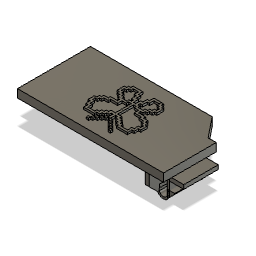
EXL-100-JOYSTICK-BATTERY-COVER (Autodesk Fusion 360 design; units mm, degrees)
Autodesk Fusion 360 part; units mm, degrees
note: some values were not read from the file. Chosen so that the rebuilt part matches the saved one: which face or edge a step refers to.
sketch "Sketch1" plane through (0, 0, 0) normal (0, 1, 0) x (1, 0, 0)
  line L0 (0, -10) -> (-30, -10)
  line L1 (-30, -10) -> (-30, 8)
  line L2 (-30, 8) -> (6, 8)
  line L3 (6, 8) -> (6, -5)
  line L4 (6, -5) -> (4, -5)
  line L5 (4, -5) -> (0, -10)
  dimension "d1" = 30
  dimension "d2" = 18
  dimension "d3" = 36
  dimension "d4" = 13
  dimension "d5" = 2
  constraint horizontal L0
  constraint perpendicular L0 L1
  constraint perpendicular L1 L2
  constraint perpendicular L2 L3
  constraint perpendicular L3 L4
  measures "d1" distance of L0.start L0.end
  measures "d2" distance of L0.end L1.end
  measures "d3" distance of L1.end L2.end
  measures "d4" distance of L2.end L3.end
  measures "d5" distance of L3.end L4.end
extrude "Extrude1" add sketch "Sketch1" along normal blind 1 makes body 1
move_body "Move1" bodies 1 to x (1, 0, 0) y (0, -1, 0) z (0, 0, -1) at (0, 0, -16)
sketch "Sketch2" plane through (0, 0, 0) normal (0, 1, 0) x (1, 0, 0)
  line L0 (105.8333, -439.2083) -> (105.8333, -418.0417)
  line L1 (105.8333, -418.0417) -> (84.6667, -418.0417)
  line L2 (84.6667, -418.0417) -> (84.6667, -460.375)
  line L3 (84.6667, -460.375) -> (107.1563, -460.375)
  line L4 (107.1563, -460.375) -> (107.1563, -481.5417)
  line L5 (107.1563, -481.5417) -> (128.451, -481.5417)
  line L6 (128.451, -481.5417) -> (128.451, -439.2083)
  line L7 (128.451, -439.2083) -> (105.8333, -439.2083)
  line L8 (283.1042, -153.4583) -> (283.1042, -132.2917)
  line L9 (283.1042, -132.2917) -> (330.7292, -132.2917)
  line L10 (330.7292, -132.2917) -> (330.7292, -153.4583)
  line L11 (330.7292, -153.4583) -> (306.9167, -153.4583)
  line L12 (306.9167, -153.4583) -> (306.9167, -174.625)
  line L13 (306.9167, -174.625) -> (264.5833, -174.625)
  line L14 (264.5833, -174.625) -> (264.5833, -153.4583)
  line L15 (264.5833, -153.4583) -> (283.1042, -153.4583)
  line L16 (42.3333, -201.0833) -> (42.3333, -221.787)
  line L17 (42.3333, -221.787) -> (63.5, -221.787)
  line L18 (63.5, -221.787) -> (63.5, -243.4167)
  line L19 (63.5, -243.4167) -> (105.8333, -243.4167)
  line L20 (105.8333, -243.4167) -> (105.8333, -264.5833)
  line L21 (105.8333, -264.5833) -> (174.625, -264.5833)
  line L22 (174.625, -264.5833) -> (174.625, -306.9167)
  line L23 (174.625, -306.9167) -> (216.9583, -306.9167)
  line L24 (216.9583, -306.9167) -> (216.9583, -328.0833)
  line L25 (216.9583, -328.0833) -> (243.4167, -328.0833)
  line L26 (243.4167, -328.0833) -> (243.4167, -174.625)
  line L27 (243.4167, -174.625) -> (201.0833, -174.625)
  line L28 (201.0833, -174.625) -> (201.0833, -153.4583)
  line L29 (201.0833, -153.4583) -> (177.2708, -153.4583)
  line L30 (177.2708, -153.4583) -> (177.2708, -132.2917)
  line L31 (177.2708, -132.2917) -> (224.8958, -132.2917)
  line L32 (224.8958, -132.2917) -> (224.8958, -153.4583)
  line L33 (224.8958, -153.4583) -> (243.4167, -153.4583)
  line L34 (243.4167, -153.4583) -> (243.4167, -105.8333)
  line L35 (243.4167, -105.8333) -> (264.5833, -105.8333)
  line L36 (264.5833, -105.8333) -> (264.5833, -328.0833)
  line L37 (264.5833, -328.0833) -> (291.0417, -328.0833)
  line L38 (291.0417, -328.0833) -> (291.0417, -306.9167)
  line L39 (291.0417, -306.9167) -> (333.375, -306.9167)
  line L40 (333.375, -306.9167) -> (333.375, -264.5833)
  line L41 (333.375, -264.5833) -> (402.1667, -264.5833)
  line L42 (402.1667, -264.5833) -> (402.1667, -243.4167)
  line L43 (402.1667, -243.4167) -> (444.5, -243.4167)
  line L44 (444.5, -243.4167) -> (444.5, -221.787)
  line L45 (444.5, -221.787) -> (465.6667, -221.787)
  line L46 (465.6667, -221.787) -> (465.6667, -201.0833)
  line L47 (465.6667, -201.0833) -> (486.8333, -201.0833)
  line L48 (486.8333, -201.0833) -> (486.8333, -174.625)
  line L49 (486.8333, -174.625) -> (465.6667, -174.625)
  line L50 (465.6667, -174.625) -> (465.6667, -132.2917)
  line L51 (465.6667, -132.2917) -> (444.5, -132.2917)
  line L52 (444.5, -132.2917) -> (444.5, -89.9583)
  line L53 (444.5, -89.9583) -> (465.6667, -89.9583)
  line L54 (465.6667, -89.9583) -> (465.6667, -111.125)
  line L55 (465.6667, -111.125) -> (486.8333, -111.125)
  line L56 (486.8333, -111.125) -> (486.8333, -153.4583)
  line L57 (486.8333, -153.4583) -> (508, -153.4583)
  line L58 (508, -153.4583) -> (508, -216.9583)
  line L59 (508, -216.9583) -> (486.8333, -216.9583)
  line L60 (486.8333, -216.9583) -> (486.8333, -242.4906)
  line L61 (486.8333, -242.4906) -> (465.6667, -242.4906)
  line L62 (465.6667, -242.4906) -> (465.6667, -264.5833)
  line L63 (465.6667, -264.5833) -> (423.3333, -264.5833)
  line L64 (423.3333, -264.5833) -> (423.3333, -285.75)
  line L65 (423.3333, -285.75) -> (354.5417, -285.75)
  line L66 (354.5417, -285.75) -> (354.5417, -306.9167)
  line L67 (354.5417, -306.9167) -> (375.7083, -306.9167)
  line L68 (375.7083, -306.9167) -> (375.7083, -328.0833)
  line L69 (375.7083, -328.0833) -> (396.875, -328.0833)
  line L70 (396.875, -328.0833) -> (396.875, -349.25)
  line L71 (396.875, -349.25) -> (423.3333, -349.25)
  line L72 (423.3333, -349.25) -> (423.3333, -370.4167)
  line L73 (423.3333, -370.4167) -> (444.5, -370.4167)
  line L74 (444.5, -370.4167) -> (444.5, -439.2083)
  line L75 (444.5, -439.2083) -> (423.3333, -439.2083)
  line L76 (423.3333, -439.2083) -> (423.3333, -391.5833)
  line L77 (423.3333, -391.5833) -> (400.8438, -391.5833)
  line L78 (400.8438, -391.5833) -> (400.8438, -370.4167)
  line L79 (400.8438, -370.4167) -> (378.3542, -370.4167)
  line L80 (378.3542, -370.4167) -> (378.3542, -349.25)
  line L81 (378.3542, -349.25) -> (354.5417, -349.25)
  line L82 (354.5417, -349.25) -> (354.5417, -328.0833)
  line L83 (354.5417, -328.0833) -> (306.9167, -328.0833)
  line L84 (306.9167, -328.0833) -> (306.9167, -349.25)
  line L85 (306.9167, -349.25) -> (285.75, -349.25)
  line L86 (285.75, -349.25) -> (285.75, -370.4167)
  line L87 (285.75, -370.4167) -> (306.9167, -370.4167)
  line L88 (306.9167, -370.4167) -> (306.9167, -418.0417)
  line L89 (306.9167, -418.0417) -> (328.0833, -418.0417)
  line L90 (328.0833, -418.0417) -> (328.0833, -460.375)
  line L91 (328.0833, -460.375) -> (379.6771, -460.375)
  line L92 (379.6771, -460.375) -> (379.6771, -439.2083)
  line L93 (379.6771, -439.2083) -> (400.8438, -439.2083)
  line L94 (400.8438, -439.2083) -> (400.8438, -418.0417)
  line L95 (400.8438, -418.0417) -> (423.3333, -418.0417)
  line L96 (423.3333, -418.0417) -> (423.3333, -460.375)
  line L97 (423.3333, -460.375) -> (400.8438, -460.375)
  line L98 (400.8438, -460.375) -> (400.8438, -481.5417)
  line L99 (400.8438, -481.5417) -> (306.9167, -481.5417)
  line L100 (306.9167, -481.5417) -> (306.9167, -439.2083)
  line L101 (306.9167, -439.2083) -> (285.75, -439.2083)
  line L102 (285.75, -439.2083) -> (285.75, -396.875)
  line L103 (285.75, -396.875) -> (264.5833, -396.875)
  line L104 (264.5833, -396.875) -> (264.5833, -349.25)
  line L105 (264.5833, -349.25) -> (243.4167, -349.25)
  line L106 (243.4167, -349.25) -> (243.4167, -396.875)
  line L107 (243.4167, -396.875) -> (222.25, -396.875)
  line L108 (222.25, -396.875) -> (222.25, -439.2083)
  line L109 (222.25, -439.2083) -> (201.0833, -439.2083)
  line L110 (201.0833, -439.2083) -> (201.0833, -481.5417)
  line L111 (201.0833, -481.5417) -> (128.451, -481.5417)
  line L112 (128.451, -481.5417) -> (128.4552, -460.375)
  line L113 (128.4552, -460.375) -> (179.9167, -460.375)
  line L114 (179.9167, -460.375) -> (179.9167, -418.0417)
  line L115 (179.9167, -418.0417) -> (201.0833, -418.0417)
  line L116 (201.0833, -418.0417) -> (201.0833, -370.4167)
  line L117 (201.0833, -370.4167) -> (222.25, -370.4167)
  line L118 (222.25, -370.4167) -> (222.25, -349.25)
  line L119 (222.25, -349.25) -> (201.0833, -349.25)
  line L120 (201.0833, -349.25) -> (201.0833, -328.0833)
  line L121 (201.0833, -328.0833) -> (153.4583, -328.0833)
  line L122 (153.4583, -328.0833) -> (153.4583, -349.25)
  line L123 (153.4583, -349.25) -> (129.6458, -349.25)
  line L124 (129.6458, -349.25) -> (129.6458, -370.4167)
  line L125 (129.6458, -370.4167) -> (107.1562, -370.4167)
  line L126 (107.1563, -370.4167) -> (107.1563, -391.5833)
  line L127 (107.1563, -391.5833) -> (84.6667, -391.5833)
  line L128 (84.6667, -391.5833) -> (84.6667, -439.2083)
  line L129 (84.6667, -439.2083) -> (63.5, -439.2083)
  line L130 (63.5, -439.2083) -> (63.5, -370.4167)
  line L131 (63.5, -370.4167) -> (84.6667, -370.4167)
  line L132 (84.6667, -370.4167) -> (84.6667, -349.25)
  line L133 (84.6667, -349.25) -> (111.125, -349.25)
  line L134 (111.125, -349.25) -> (111.125, -328.0833)
  line L135 (111.125, -328.0833) -> (132.2917, -328.0833)
  line L136 (132.2917, -328.0833) -> (132.2917, -306.9167)
  line L137 (132.2917, -306.9167) -> (153.4583, -306.9167)
  line L138 (153.4583, -306.9167) -> (153.4583, -285.75)
  line L139 (153.4583, -285.75) -> (84.6667, -285.75)
  line L140 (84.6667, -285.75) -> (84.6667, -264.5833)
  line L141 (84.6667, -264.5833) -> (42.3333, -264.5833)
  line L142 (42.3333, -264.5833) -> (42.3333, -242.4906)
  line L143 (42.3333, -242.4906) -> (21.1667, -242.4906)
  line L144 (21.1667, -242.4906) -> (21.1667, -216.9583)
  line L145 (21.1667, -216.9583) -> (0, -216.9583)
  line L146 (0, -216.9583) -> (0, -153.4583)
  line L147 (0, -153.4583) -> (21.1667, -153.4583)
  line L148 (21.1667, -153.4583) -> (21.1667, -111.125)
  line L149 (21.1667, -111.125) -> (42.3333, -111.125)
  line L150 (42.3333, -111.125) -> (42.3333, -89.9583)
  line L151 (42.3333, -89.9583) -> (63.5, -89.9583)
  line L152 (63.5, -89.9583) -> (63.5, -132.2917)
  line L153 (63.5, -132.2917) -> (42.3333, -132.2917)
  line L154 (42.3333, -132.2917) -> (42.3333, -174.625)
  line L155 (42.3333, -174.625) -> (21.1667, -174.625)
  line L156 (21.1667, -174.625) -> (21.1667, -201.0833)
  line L157 (21.1667, -201.0833) -> (42.3333, -201.0833)
  line L158 (359.8333, -89.9583) -> (359.8333, -68.7917)
  line L159 (359.8333, -68.7917) -> (465.6667, -68.7917)
  line L160 (465.6667, -68.7917) -> (465.6667, -89.9583)
  line L161 (465.6667, -89.9583) -> (378.3542, -89.9583)
  line L162 (378.3542, -89.9583) -> (378.3542, -111.125)
  line L163 (378.3542, -111.125) -> (354.5417, -111.125)
  line L164 (354.5417, -111.125) -> (354.5417, -132.2917)
  line L165 (354.5417, -132.2917) -> (306.9167, -132.2917)
  line L166 (306.9167, -132.2917) -> (306.9167, -111.125)
  line L167 (306.9167, -111.125) -> (330.7292, -111.125)
  line L168 (330.7292, -111.125) -> (330.7292, -89.9583)
  line L169 (330.7292, -89.9583) -> (359.8333, -89.9583)
  line L170 (42.3333, -89.9583) -> (129.6458, -89.9583)
  line L171 (129.6458, -89.9583) -> (129.6458, -111.125)
  line L172 (129.6458, -111.125) -> (153.4583, -111.125)
  line L173 (153.4583, -111.125) -> (153.4583, -132.2917)
  line L174 (153.4583, -132.2917) -> (201.0833, -132.2917)
  line L175 (201.0833, -132.2917) -> (201.0833, -111.125)
  line L176 (201.0833, -111.125) -> (177.2708, -111.125)
  line L177 (177.2708, -111.125) -> (177.2708, -89.9583)
  line L178 (177.2708, -89.9583) -> (148.1667, -89.9583)
  line L179 (148.1667, -89.9583) -> (148.1667, -68.7917)
  line L180 (148.1667, -68.7917) -> (42.3333, -68.7917)
  line L181 (42.3333, -68.7917) -> (42.3333, -89.9583)
  line L182 (285.75, -84.6667) -> (264.5833, -84.6667)
  line L183 (264.5833, -84.6667) -> (264.5833, -105.8333)
  line L184 (264.5833, -105.8333) -> (285.75, -105.8333)
  line L185 (285.75, -105.8333) -> (285.75, -84.6667)
  line L186 (243.4167, -84.6667) -> (222.25, -84.6667)
  line L187 (222.25, -84.6667) -> (222.25, -105.8333)
  line L188 (222.25, -105.8333) -> (243.4167, -105.8333)
  line L189 (243.4167, -105.8333) -> (243.4167, -84.6667)
  line L190 (179.9167, -63.5) -> (201.0833, -63.5)
  line L191 (201.0833, -63.5) -> (201.0833, -84.6667)
  line L192 (201.0833, -84.6667) -> (222.25, -84.6667)
  line L193 (222.25, -84.6667) -> (222.25, -63.5)
  line L194 (222.25, -63.5) -> (201.0833, -63.5)
  line L195 (201.0833, -63.5) -> (201.0833, -42.3333)
  line L196 (201.0833, -42.3333) -> (179.9167, -42.3333)
  line L197 (179.9167, -42.3333) -> (179.9167, -63.5)
  line L198 (306.9167, -63.5) -> (285.75, -63.5)
  line L199 (285.75, -63.5) -> (285.75, -84.6667)
  line L200 (285.75, -84.6667) -> (306.9167, -84.6667)
  line L201 (306.9167, -84.6667) -> (306.9167, -63.5)
  line L202 (328.0833, -42.3333) -> (306.9167, -42.3333)
  line L203 (306.9167, -42.3333) -> (306.9167, -63.5)
  line L204 (306.9167, -63.5) -> (328.0833, -63.5)
  line L205 (328.0833, -63.5) -> (328.0833, -42.3333)
  line L206 (179.9167, -21.1667) -> (158.75, -21.1667)
  line L207 (158.75, -21.1667) -> (158.75, -42.3333)
  line L208 (158.75, -42.3333) -> (179.9167, -42.3333)
  line L209 (179.9167, -42.3333) -> (179.9167, -21.1667)
  line L210 (349.25, -21.1667) -> (328.0833, -21.1667)
  line L211 (328.0833, -21.1667) -> (328.0833, -42.3333)
  line L212 (328.0833, -42.3333) -> (349.25, -42.3333)
  line L213 (349.25, -42.3333) -> (349.25, -21.1667)
  line L214 (370.4167, 0) -> (349.25, 0)
  line L215 (349.25, 0) -> (349.25, -21.1667)
  line L216 (349.25, -21.1667) -> (370.4167, -21.1667)
  line L217 (370.4167, -21.1667) -> (370.4167, 0)
  line L218 (158.75, 0) -> (137.5833, 0)
  line L219 (137.5833, 0) -> (137.5833, -21.1667)
  line L220 (137.5833, -21.1667) -> (158.75, -21.1667)
  line L221 (158.75, -21.1667) -> (158.75, 0)
extrude "Extrude2" add sketch "Sketch2" along normal blind 0.5 separate body contours L0 L1 L2 L3 L4 L5 L6 L7 L128 | L2 L14 L16 L17 L18 L19 L20 L21 L22 L23 L24 L25 L26 L27 L28 L29 L30 L31 L32 L33 L34 L35 L36 L37 L38 L39 L40 L41 L42 L43 L44 L45 L46 L47 L48 L49 L50 L51 L52 L53 L54 L55 L56 L57 L58 L59 L60 L61 L62 L63 L64 L65 L66 L67 L68 L69 L70 L71 L72 L73 L74 L75 L96 L97 L98 L99 L100 L101 L102 L103 L104 L105 L106 L107 L108 L109 L110 L111 L112 L113 L114 L115 L116 L117 L118 L119 L120 L121 L122 L123 L124 L125 L126 L127 L128 L129 L130 L131 L132 L133 L134 L135 L136 L137 L138 L139 L140 L141 L142 L143 L144 L145 L146 L147 L148 L149 L150 L151 L152 L153 L154 L155 L156 L157 L161 L170 L174 | L218 L219 L220 L221 | L206 L207 L208 L209 | L190 L195 L196 L197 | L191 L192 L193 L194 | L186 L187 L188 L189 | L214 L215 L216 L217 | L210 L211 L212 L213 | L202 L203 L204 L205 | L198 L199 L200 L201 | L182 L183 L184 L185 | L31 L151 L170 L171 L172 L173 L174 L175 L176 L177 L178 L179 L180 L181 | L8 L9 L10 L11 L12 L13 L14 L15 L36 L165 | L9 L53 L158 L159 L160 L161 L162 L163 L164 L165 L166 L167 L168 L169 makes body 2 at (84.6667, 0.5, 75.8472)
scale "Scale1" factors (0.2, 1, 0.2) about (243.4167, 0, 174.625) bodies 2
move_body "Move2" bodies 2 to x (1, 0, 0) y (0, 1, 0) z (0, 0, 1) at (-239.4762, 0, -125.5632)
scale "Scale2" factors (0.2, 1, 0.2) about (8.1738, 0, 49.0618) bodies 2
move_body "Move3" bodies 2 to x (1, 0, 0) y (0, 1, 0) z (0, 0, 1) at (-21.1687, 0, -68.5097)
scale "Scale3" factors (0.639764, 1, 0.639764) about (-12.995, 0, -19.448) bodies 2
move_body "Move4" bodies 2 to x (1, 0, 0) y (0, 1, 0) z (0, 0, 1) at (0, 0, 23.8705)
move_body "Move5" bodies 2 to x (-1, 0, 0) y (0, 1, 0) z (0, 0, -1) at (-39.5316, 0, 8.7893)
move_body "Align1" bodies 2 to x (1, 0, 0) y (0, 1, 0) z (0, 0, 1) at (14.2658, 0, -18.7938)
box "BoxPrimitive1" add length 5 width 13 height 2 placed x (0, 0, 1) y (1, 0, 0) z (0, 1, 0) at (-45, 0, -5) separate body makes body 3
move_body "Move6" bodies 3 to x (0, 0, 1) y (0, 1, 0) z (-1, 0, 0) at (-50, 0, 40)
move_body "Align2" bodies 3 to x (1, 0, 0) y (0, -1, 0) z (0, 0, -1) at (20, 1, -15.5)
move_body "Move7" bodies 3 to x (1, 0, 0) y (0, 1, 0) z (0, 0, 1) at (0, -2, 0)
move_body "Move8" bodies 3 to x (1, 0, 0) y (0, 1, 0) z (0, 0, 1) at (-2, 0, 0)
chamfer "Chamfer1" distance 2 angle 45 1 edges at (-27, -3, -17) on bodies 3
box "BoxPrimitive2" add length 15 width 1 height 10 placed x (0, 0, 1) y (1, 0, 0) z (0, 1, 0) at (3, 0, -3) separate body makes body 4
move_body "Align3" bodies 4 to x (1, 0, 0) y (0, -1, 0) z (0, 0, -1) at (2, 9, -10)
move_body "Move9" bodies 4 to x (1, 0, 0) y (0, 1, 0) z (0, 0, 1) at (-2, 0, 0)
move_face "MoveFace1" by (0, 0, 1) 1 faces at (3.3333, 5.6667, -22) on bodies 4
move_face "MoveFace2" by (0, 0, -1) 1 faces at (3.3333, 5.6667, -7) on bodies 4
move_body "Move10" bodies 4 to x (1, 0, 0) y (0, 1, 0) z (0, 0, 1) at (0, -10, 0)
box "BoxPrimitive3" add length 2 width 2 height 13 placed x (0, 1, 0) y (-1, 0, 0) z (0, 0, 1) at (6, -11, 0) separate body makes body 5
move_body "Align4" bodies 5 to x (0, 0, 1) y (0, 1, 0) z (-1, 0, 0) at (4, 0, -25)
move_body "Move11" bodies 5 to x (0, 0, -1) y (0, 1, 0) z (1, 0, 0) at (25, 0, -17)
chamfer "Chamfer2" distance 2 angle 45 1 edges at (6, -11, -14.5) on bodies 5
move_body "Move12" bodies 2 to x (1, 0, 0) y (0, 1, 0) z (0, 0, 1) at (0, 1, 0)
move_face "MoveFace3" by (0, 1, 0) 1 faces at (-20, 0, -20) on bodies 1
move_face "MoveFace4" by (0, -2, 0) 1 faces at (3.6667, -1, -12.3333) on bodies 4
move_body "Move13" bodies 4 5 to x (1, 0, 0) y (0, 1, 0) z (0, 0, 1) at (0, 2, 0)
combine "Combine1" operation add target body 1 tool bodies 3 4 5 2 keep tools result as body 6 in component "Component"
move_face "MoveFace5" by (0, -2.5, 0) 1 faces at (3.6667, -1, -12.3333) on bodies 4
move_body "Move14" bodies 4 5 to x (1, 0, 0) y (0, 1, 0) z (0, 0, 1) at (0, 2.5, 0)
sketch "Sketch6" plane through (0, 0, 0) normal (0, 0, 1) x (1, 0, 0)
  line L0 (5.8145, -7.1066) -> (5.8145, -2)
  constraint vertical L0
split "Split1" by curves path "Sketch6" along L0 bodies 5 makes body 7 at (5.9382, -4.5622, -16.6667)
delete_body "RemoveBody1" bodies 7
combine "Combine1'" operation add target body 1 tool bodies 3 4 5 2 keep tools result as body 8 in component "Component'"
copy_body "CopyPasteBodies1" bodies 4 5 makes body 9 makes body 10
move_body "Move15" bodies 9 10 to x (1, 0, 0) y (0, 1, 0) z (0, 0, 1) at (0, 0, 0)
box "BoxPrimitive4" add length 9 width 2 height 2 placed x (0, 0, -1) y (-1, 0, 0) z (0, 1, 0) at (9, 0, -12) separate body makes body 11
move_body "Align5" bodies 11 to x (1, 0, 0) y (0, -1, 0) z (0, 0, -1) at (-1, 3, -31)
move_body "Move16" bodies 11 to x (1, 0, 0) y (0, 1, 0) z (0, 0, 1) at (0, -4, 0)
move_body "Move17" bodies 10 to x (1, 0, 0) y (0, 1, 0) z (0, 0, 1) at (2, 0, 0)
sketch "Sketch8" plane through (0, 0, 0) normal (0, 0, 1) x (1, 0, 0)
cylinder "CylinderPrimitive1" add diameter 3 height 13 placed x (1, 0, 0) y (0, 1, 0) z (0, 0, 1) at (3.5, -7.5, 0) separate body makes body 12
move_body "Move18" bodies 12 to x (1, 0, 0) y (0, 1, 0) z (0, 0, 1) at (0.943, 1.066, 0)
box "BoxPrimitive5" add length 3.884 width 1 height 13 placed x (0, -1, 0) y (1, 0, 0) z (0, 0, 1) at (10, -3, 0) separate body makes body 13
move_face "MoveFace6" by (0, 0, -4) 1 faces at (10.6667, -4.2947, 13) on bodies 13
move_body "Align6" bodies 13 to x (1, 0, 0) y (0, -1, 0) z (0, 0, -1) at (-5, -5, -10)
move_body "Move19" bodies 13 to x (1, 0, 0) y (0, 1, 0) z (0, 0, 1) at (0, -2.8795, 0)
move_body "Move20" bodies 12 to x (1, 0, 0) y (0, 1, 0) z (0, 0, 1) at (0, 0, -13)
move_body "Move21" bodies 12 to x (1, 0, 0) y (0, 1, 0) z (0, 0, 1) at (0, 0, -7.9922)
move_face "MoveFace7" by (0, 0, -2) 1 faces at (4.6609, -6.105, -7.9922) on bodies 12
move_face "MoveFace8" by (0, 0, 2) 1 faces at (5.0101, -6.9722, -20.9922) on bodies 12
move_face "MoveFace9" by (0, -2.9383, 0) 1 faces at (5.3333, -4.8795, -13) on bodies 13
move_body "Move22" bodies 12 to x (1, 0, 0) y (0, 1, 0) z (0, 0, 1) at (0, -1.1166, 0)
move_body "Move23" bodies 10 to x (1, 0, 0) y (0, 1, 0) z (0, 0, 1) at (-0.94, 0, 0)
move_face "MoveFace10" by (-0.496, 0, 0) 1 faces at (6.8745, -4.6239, -16.6667) on bodies 10
move_face "MoveFace11" by (0, -1.2772, 0) 1 faces at (3.6667, -6.5, -12.3333) on bodies 9
chamfer "Chamfer3" distance 2.026 angle 45 1 edges at (3.5, -7.7772, -21) on bodies 9
chamfer "Chamfer4" distance 2.058 angle 45 1 edges at (3.5, -7.7772, -8) on bodies 9
combine "Combine1''" operation add target body 9 tool bodies 13 12 11 10 1 2 3 keep tools result as body 14 in component "Component''"
cylinder "CylinderPrimitive2" add diameter 2 height 15 placed x (1, 0, 0) y (0, 1, 0) z (0, 0, 1) at (-3, -10, 0) separate body makes body 15
move_body "Align7" bodies 15 to x (1, 0, 0) y (0, 1, 0) z (0, 0, 1) at (7.443, 2.4495, -18.9922)
combine "Combine1'''" operation cut target body 12 tool bodies 15
box "BoxPrimitive6" add length 4.31 width 1.916 height 13 placed x (0, 1, 0) y (-1, 0, 0) z (0, 0, 1) at (5.4365, -9.8355, 0) separate body makes body 16
move_body "Move24" bodies 16 to x (1, 0, 0) y (0, 1, 0) z (0, 0, 1) at (0, 2.1552, 0)
move_body "Move25" bodies 16 to x (1, 0, 0) y (0, 1, 0) z (0, 0, 1) at (0, 0, -21.0732)
combine "Combine2" operation cut target body 12 tool bodies 16
combine "Combine1''''" operation add target body 9 tool bodies 13 12 11 10 1 2 3 keep tools result as body 17 in component "Component'''"
move_face "MoveFace12" by (0, -0.5, 0) 1 faces at (5.3333, -0.9955, -13) on bodies 13
move_face "MoveFace13" by (0, -0.5, 0) 1 faces at (6.6667, -1, -16) on bodies 11
move_face "MoveFace14" by (0.5, 0, 0) 1 faces at (8, -2, -13) on bodies 11
combine "Combine1'''''" operation add target body 1 tool bodies 3 2 9 10 11 12 13 keep tools result as body 18 in component "Component''''"
move_body "Move26" bodies 9 13 12 11 10 to x (1, 0, 0) y (0, 1, 0) z (0, 0, 1) at (-0.5, 0, 0)
move_face "MoveFace15" by (0.5, 0, 0) 1 faces at (5.8785, -4.9546, -16.6667) on bodies 10
move_face "MoveFace16" by (0, 0, -2) 1 faces at (5.1663, -5.2273, -8) on bodies 10
move_face "MoveFace17" by (0, 0, 2) 1 faces at (5.1663, -5.2273, -21) on bodies 10
move_face "MoveFace18" by (0.5, 0, 0) 1 faces at (8, -2, -13) on bodies 11
combine "Combine1''''''" operation add target body 9 tool bodies 13 12 11 10 1 2 3 keep tools result as body 19 in component "Component'''''"
move_body "Move27" bodies 9 to x (1, 0, 0) y (0, 1, 0) z (0, 0, 1) at (-1, 0, 0)
move_body "Move28" bodies 12 to x (1, 0, 0) y (0, 1, 0) z (0, 0, 1) at (-0.5, 0, 0)
move_body "Move29" bodies 13 11 10 to x (1, 0, 0) y (0, 1, 0) z (0, 0, 1) at (-0.5, 0, 0)
move_face "MoveFace19" by (0.5, 0, 0) 1 faces at (8, -2, -13) on bodies 11
combine "Combine1'''''''" operation add target body 1 tool bodies 3 13 12 11 2 9 10 keep tools result as body 20 in component "Component''''''"
move_body "Move30" bodies 10 to x (1, 0, 0) y (0, 1, 0) z (0, 0, 1) at (0.5, 0, 0)
move_body "Move31" bodies 10 to x (1, 0, 0) y (0, 1, 0) z (0, 0, 1) at (-0.4, 0, 0)
move_face "MoveFace20" by (0, 0.5, 0) 1 faces at (6.1667, -3, -16) on bodies 11
combine "Combine1''''''''" operation add target body 1 tool bodies 3 13 12 11 2 9 10 keep tools result as body 21 in component "Component'''''''"
move_body "Move32" bodies 12 to x (1, 0, 0) y (0, 1, 0) z (0, 0, 1) at (0, 2, 0)
move_face "MoveFace21" by (0, 2, 0) 5 faces at (2.1667, -7.7772, -13.03) (2.1667, -6.4052, -8.686) (1.8333, -6.4265, -20.3247) (2.1667, -4.1461, -8) (2.1667, -4.1674, -21) on bodies 9
move_face "MoveFace22" by (0, 2, 0) 1 faces at (4.3333, -7.8178, -13) on bodies 13
move_body "Move33" bodies 10 to x (1, 0, 0) y (0, 1, 0) z (0, 0, 1) at (0.3, 0, 0)
move_face "MoveFace23" by (0.4267, 0, 0) 3 faces at (4.3333, -5.8178, -13) (4, -4.3771, -13) (4.3333, -1.4955, -13) on bodies 13
combine "Combine1'''''''''" operation add target body 1 tool bodies 3 13 12 11 2 9 10 keep tools result as body 22 in component "Component''''''''"
move_face "MoveFace24" by (0, 0, -0.5) 1 faces at (7.3333, -1.8333, -10) on bodies 11
move_face "MoveFace25" by (0, 0, -0.5) 1 faces at (4.8089, -4.3771, -10) on bodies 13
move_face "MoveFace26" by (0, 0, -0.5) 2 faces at (5.0663, -5.2273, -10) (2.2128, -5.0436, -9.9922) on bodies 10 12
chamfer "Chamfer5" distance 0.542 angle 45 1 edges at (4.4267, -1.4955, -14.75) on bodies 13
combine "Combine1''''''''''" operation add target body 1 tool bodies 3 13 12 11 2 9 10 keep tools result as body 23 in component "EXL-100-JOYSTICK-BATTERY-DOOR"
component "EXL-100-JOYSTICK-BATTERY-DOOR" placed x (1, 0, 0) y (0, 1, 0) z (0, 0, 1) at (0, 0, 0)
named bodies: "Main", "Icon", "Hinge", "Lock-Stem-No-Spring-Lock", "Lock-Bolt-No-Spring-Lock", "Lock-Bolt (1)", "Lock-Stem", "Lock-Bolt", "Lock-Stem-Spring-Lock", "Lock-Bolt-Spring-Lock", "Lock-Handle-Spring-Lock", "Lock-Handle-Spring-Spring-Lock", "Lock-Handle-Guide", "Lock-Stem (1)"
